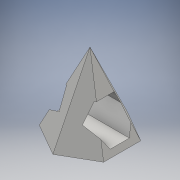
# Autodesk Inventor part: пирамида
Saved by Autodesk Inventor 2016 (Build 200138000, 138)
## iProperties
Created: 2016-10-05
Part Number: пирамида
Material: Типовые
Document SubType Name: Modeling
Designer: Student
Density: 1 g/cm^3
Appearance: По умолчанию
Mass: 14.1318 g
Surface Area: 66.4661 cm^2
Volume: 14.1318 cm^3
Author: Student
Autodesk Inventor part; units mm, degrees
ref_plane "XZ Plane" through (0, 0, 0) normal (0, 1, 0) x (-1, 0, 0)
sketch "Эскиз1" plane through (0, 0, 0) normal (0, 0, 1) x (1, 0, 0)
  line L0 (0, -25) -> (-21.6506, -12.5)
  line L1 (-21.6506, -12.5) -> (-21.6506, 12.5)
  line L2 (-21.6506, 12.5) -> (0, 25)
  line L3 (0, 25) -> (21.6506, 12.5)
  line L4 (21.6506, 12.5) -> (21.6506, -12.5)
  line L5 (21.6506, -12.5) -> (0, -25)
  point P0 (0, 0)
  point P1 (0, 0)
  constraints: 12 end point, 13 other
ref_plane "РабПлоскость1" through (0, 0, 50) normal (0, 0, 1) x (1, 0, 0)
sketch "Эскиз2" plane through (0, 0, 50) normal (0, 0, 1) x (1, 0, 0)
  point P0 (0, 0)
  point P1 (0, 0)
  constraints: 1 coincident
loft "Лофт1" add profiles "Эскиз1" section 2 point at (0, 0, 50)
ref_plane "РабПлоскость2" through (25, 0, 0) normal (1, 0, 0) x (0, 1, 0)
sketch "Эскиз3" plane through (25, 0, 0) normal (1, 0, 0) x (0, 1, 0)
  line L0 (25, 0) -> (0, 50) projected
  line L1 (13, 15) -> (6.5, 3.7417)
  line L2 (6.5, 3.7417) -> (-6.5, 3.7417)
  line L3 (-6.5, 3.7417) -> (-13, 15)
  line L4 (-13, 15) -> (-6.5, 26.2583)
  line L5 (-6.5, 26.2583) -> (6.5, 26.2583)
  line L6 (6.5, 26.2583) -> (13, 15)
  point P0 (0, 0)
  point P1 (0, 15)
  constraints: 12 end point, 13 other
extrude "Выдавливание1" cut sketch "Эскиз3" against normal blind 50
